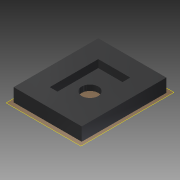
# Autodesk Inventor part: InlayOben
Saved by Autodesk Inventor 2014 (Build 180170000, 170)
## iProperties
Created: 2016-09-06
Part Number: InlayOben
Material: Gummi, Silikon
Document SubType Name: Modeling
Designer: cem
Density: 1 g/cm^3
Appearance: Gummi - schwarz - Version 1.1
Author: cem
Autodesk Inventor part; units mm, degrees
ref_plane "YZ Plane" through (0, 0, 0) normal (1, 0, 0) x (0, 1, 0)
ref_plane "XZ Plane" through (0, 0, 0) normal (0, 1, 0) x (-1, 0, 0)
ref_plane "XY Plane" through (0, 0, 0) normal (0, 0, 1) x (1, 0, 0)
ref_plane "Arbeitsebene1" through (0, 0, 0) normal (0, 0, 1) x (1, 0, 0)
sketch "Skizze1" plane through (0, 0, 0) normal (0, 0, 1) x (1, 0, 0)
  line L0 (-28.4, 40.9) -> (28.4, 40.9) projected
  line L1 (28.4, 40.9) -> (28.4, -40.9) projected
  line L2 (28.4, -40.9) -> (-28.4, -40.9) projected
  line L3 (-28.4, -40.9) -> (-28.4, 40.9) projected
  line L4 (-33.4, 45.9) -> (-33.4, -45.9) projected
  line L5 (-33.4, -45.9) -> (33.4, -45.9) projected
  line L6 (33.4, -45.9) -> (33.4, 45.9) projected
  line L7 (33.4, 45.9) -> (-33.4, 45.9) projected
  line L8 (-28.4, 40.9) -> (28.4, 40.9) projected
  line L9 (28.4, 40.9) -> (28.4, -40.9) projected
  line L10 (28.4, -40.9) -> (-28.4, -40.9) projected
  line L11 (-28.4, -40.9) -> (-28.4, 40.9) projected
  line L12 (-33.4, 45.9) -> (-33.4, -45.9) projected
  line L13 (-33.4, -45.9) -> (33.4, -45.9) projected
  line L14 (33.4, -45.9) -> (33.4, 45.9) projected
  line L15 (33.4, 45.9) -> (-33.4, 45.9) projected
  point P0 (0, 0)
extrude "Extrusion1" add sketch "Skizze1" along normal blind 5 contours L0 L1 L2 L3 | L7 L6 L5 L4
sketch "Skizze2" plane through (0, 0, 5) normal (0, 0, 1) x (1, 0, 0)
  circle A0 centre (0, 0) radius 7.5
  dimension "d2" = 15
  constraints: 1 centre point, 1 coincident
  measures "d2" diameter of A0
extrude "Extrusion2" cut sketch "Skizze2" against normal up to next
sketch "Skizze3" plane through (0, 0, 5) normal (0, 0, 1) x (1, 0, 0)
  line L0 (-33.4, 45.9) -> (-33.4, -45.9) projected
  line L1 (-33.4, -45.9) -> (33.4, -45.9) projected
  line L2 (33.4, -45.9) -> (33.4, 45.9) projected
  line L3 (33.4, 45.9) -> (-33.4, 45.9) projected
  line L4 (-14.5, 22) -> (14.5, 22)
  line L5 (14.5, 22) -> (14.5, -22)
  line L6 (14.5, -22) -> (-14.5, -22)
  line L7 (-14.5, -22) -> (-14.5, 22)
  line L8 (0, -64.26) -> (0, 64.26) projected
  line L9 (-46.76, 0) -> (46.76, 0) projected
  dimension "d9" = 29
  dimension "d10" = 44
  constraints: 8 end point, 2 parallel, 1 horizontal, 1 perpendicular, 2 other
  measures "d9" distance between parallel lines of L5 L7
  measures "d10" distance between parallel lines of L6 L4
extrude "Extrusion4" add sketch "Skizze3" along normal blind 7 contours L3 L8 L4 L7 L9 L0 | L9 L7 L6 L8 L1 L0 | L3 L2 L9 L5 L4 L8 | L8 L6 L5 L9 L2 L1
